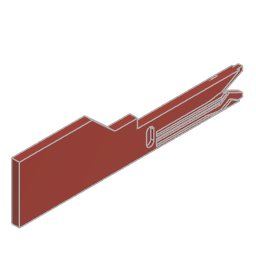
3ks+ finished (Autodesk Fusion 360 design; units mm, degrees)
Autodesk Fusion 360 part; units mm, degrees
note: some values were not read from the file. Set by a fixed rule: which face or edge a step refers to.
sketch "blade" plane through (0, 0, 0) normal (1, 0, 0) x (0, 1, 0)
  line L0 (0, 0) -> (0, 0.75) construction
  line L1 (0, 0.75) -> (25.25, 0.75)
  line L2 (25.25, 0.75) -> (25.25, 8.75)
  line L3 (25.25, 8.75) -> (0, 8.75)
  line L4 (0, 8.75) -> (0, 0.75)
  dimension "d14" = 0.75
  dimension "d15" = 25.25
  dimension "d16" = 8
  constraint coincident L0.start origin
  constraint vertical L0
  constraint horizontal L1
  constraint vertical L2
  constraint horizontal L3
  constraint vertical L4
  measures "d14" distance of L0.start L0.end
  measures "d15" distance of L0.end L1.end
  measures "d16" distance of L0.end L3.end
extrude "Extrude1" add sketch "blade" along normal blind 1.1 makes body 1
sketch "single track" plane through (1.1, 0, 0) normal (1, 0, 0) x (0, 1, 0)
  line L0 (0, 8.75) -> (0, 0.75)
  line L1 (0, 0.75) -> (25.25, 0.75)
  line L2 (25.25, 0.75) -> (25.25, 8.75)
  line L3 (25.25, 8.75) -> (0, 8.75)
  line L4 (0, 0.75) -> (0.9, 0.75) construction
  line L5 (0.9, 0.75) -> (4.4, 0.75) construction
  line L6 (4.4, 0.75) -> (7.9, 0.75) construction
  line L7 (7.9, 0.75) -> (11.4, 0.75) construction
  line L8 (11.4, 0.75) -> (14.9, 0.75) construction
  line L9 (14.9, 0.75) -> (18.4, 0.75) construction
  line L10 (18.4, 0.75) -> (21.9, 0.75) construction
  line L11 (21.9, 0.75) -> (21.9, 4.75) construction
  line L12 (21.9, 4.75) -> (25.25, 4.75)
  line L13 (0.9, 0.75) -> (0.9, 2.75) construction
  line L14 (4.4, 0.75) -> (4.4, 2.75) construction
  line L15 (7.9, 0.75) -> (7.9, 2.75) construction
  line L16 (11.4, 0.75) -> (11.4, 2.75) construction
  line L17 (14.9, 0.75) -> (14.9, 2.75) construction
  line L18 (18.4, 0.75) -> (18.4, 2.75) construction
  circle A0 centre (0.9, 2.75) radius 0.6 construction
  circle A1 centre (4.4, 2.75) radius 0.6 construction
  circle A2 centre (7.9, 2.75) radius 0.6 construction
  circle A3 centre (11.4, 2.75) radius 0.6 construction
  circle A4 centre (14.9, 2.75) radius 0.6 construction
  circle A5 centre (18.4, 2.75) radius 0.6 construction
  line L19 (0.9, 2.75) -> (0, 2.75)
  line L20 (0, 0.75) -> (0, 2.75) construction
  line L21 (0.9, 2.75) -> (1.2, 2.75)
  line L22 (4.4, 2.75) -> (4.1, 2.75)
  line L23 (4.4, 2.75) -> (4.7, 2.75)
  line L24 (7.9, 2.75) -> (7.6, 2.75)
  line L25 (7.9, 2.75) -> (8.2, 2.75)
  line L26 (11.4, 2.75) -> (11.1, 2.75)
  line L27 (11.4, 2.75) -> (11.7, 2.75)
  line L28 (14.9, 2.75) -> (14.6, 2.75)
  line L29 (14.9, 2.75) -> (15.2, 2.75)
  line L30 (18.4, 2.75) -> (18.1, 2.75)
  line L31 (18.4, 2.75) -> (18.7, 2.75)
  line L32 (21.9, 4.75) -> (21.6, 4.75)
  line L33 (1.2, 2.75) -> (4.1, 2.75)
  line L34 (4.7, 2.75) -> (7.6, 2.75)
  line L35 (8.2, 2.75) -> (11.1, 2.75)
  line L36 (11.7, 2.75) -> (14.6, 2.75)
  line L37 (15.2, 2.75) -> (18.1, 2.75)
  line L38 (18.7, 2.75) -> (21.6, 4.75)
  dimension "d19" = 0.9
  dimension "d20" = 3.5
  dimension "d21" = 3.5
  dimension "d22" = 3.5
  dimension "d23" = 3.5
  dimension "d24" = 3.5
  dimension "d25" = 3.5
  dimension "d26" = 2
  dimension "d27" = 2
  dimension "d28" = 2
  dimension "d29" = 2
  dimension "d30" = 2
  dimension "d31" = 2
  dimension "d32" = 1.2
  dimension "d33" = 1.2
  dimension "d34" = 1.2
  dimension "d35" = 1.2
  dimension "d36" = 1.2
  dimension "d37" = 1.2
  dimension "d38" = 0.3
  dimension "d39" = 0.3
  dimension "d40" = 0.3
  dimension "d41" = 0.3
  dimension "d42" = 0.3
  dimension "d43" = 0.3
  dimension "d44" = 0.3
  dimension "d45" = 0.3
  dimension "d46" = 0.3
  dimension "d47" = 0.3
  dimension "d48" = 0.3
  dimension "d49" = 0.3
  constraint coincident L0.end L1.start
  constraint perpendicular L0 L4
  constraint parallel L1 L5
  constraint parallel L1 L6
  constraint parallel L1 L7
  constraint parallel L1 L8
  constraint parallel L1 L9
  constraint parallel L1 L10
  constraint perpendicular L10 L11
  constraint midpoint L2 L12.end
  constraint perpendicular L2 L12
  constraint perpendicular L5 L13
  constraint perpendicular L6 L14
  constraint perpendicular L6 L15
  constraint perpendicular L8 L16
  constraint perpendicular L9 L17
  constraint perpendicular L9 L18
  constraint coincident L13.end A0.centre
  constraint coincident L14.end A1.centre
  constraint coincident L15.end A2.centre
  constraint coincident L16.end A3.centre
  constraint coincident L17.end A4.centre
  constraint coincident L18.end A5.centre
  constraint coincident L0 L19.end
  constraint perpendicular L0 L19
  constraint perpendicular L13 L21
  constraint perpendicular L14 L22
  constraint perpendicular L14 L23
  constraint perpendicular L15 L24
  constraint perpendicular L15 L25
  constraint perpendicular L16 L26
  constraint perpendicular L16 L27
  constraint perpendicular L17 L28
  constraint perpendicular L17 L29
  constraint perpendicular L18 L30
  constraint perpendicular L18 L31
  constraint perpendicular L11 L32
  measures "d19" distance of L0.end L4.end
  measures "d20" distance of L4.end L5.end
  measures "d21" distance of L5.end L6.end
  measures "d22" distance of L6.end L7.end
  measures "d23" distance of L7.end L8.end
  measures "d24" distance of L8.end L9.end
  measures "d25" distance of L9.end L10.end
  measures "d26" distance of L4.end L13.end
  measures "d27" distance of L5.end L14.end
  measures "d28" distance of L6.end L15.end
  measures "d29" distance of L7.end L16.end
  measures "d30" distance of L8.end L17.end
  measures "d31" distance of L9.end L18.end
  measures "d32" diameter of A0
  measures "d33" diameter of A1
  measures "d34" diameter of A2
  measures "d35" diameter of A3
  measures "d36" diameter of A4
  measures "d37" diameter of A5
  measures "d38" distance of L13.end L21.end
  measures "d39" distance of L14.end L22.end
  measures "d40" distance of L14.end L23.end
  measures "d41" distance of L15.end L24.end
  measures "d42" distance of L15.end L25.end
  measures "d43" distance of L16.end L26.end
  measures "d44" distance of L16.end L27.end
  measures "d45" distance of L17.end L28.end
  measures "d46" distance of L17.end L29.end
  measures "d47" distance of L18.end L30.end
  measures "d48" distance of L18.end L31.end
  measures "d49" distance of L11.end L32.end
sketch "single track cutter" plane through (0, 0, 0) normal (0, -1, 0) x (1, 0, 0)
  line L0 (0, 8.75) -> (0, 0.75)
  line L1 (0, 0.75) -> (1.1, 0.75)
  line L2 (1.1, 0.75) -> (1.1, 8.75)
  line L3 (1.1, 8.75) -> (0, 8.75)
  line L4 (1.1, 2.75) -> (1.1, 2.15)
  line L5 (1.1, 2.75) -> (1.1, 3.35)
  line L6 (1.1, 3.35) -> (0.1, 3.35)
  line L7 (0.1, 3.35) -> (0.1, 2.15)
  line L8 (0.1, 2.15) -> (1.1, 2.15)
  point P0 (1.1, 2.75)
  dimension "d50" = 0.6
  dimension "d51" = 0.6
  dimension "d52" = 1
  constraint vertical L4
  constraint coincident P0 L4.start
  constraint parallel L2 L5
  constraint perpendicular L5 L6
  constraint perpendicular L6 L7
  constraint perpendicular L4 L8
  measures "d50" distance of P0 L4.end
  measures "d51" distance of P0 L5.end
  measures "d52" distance of L5.end L6.end
sketch "double track" plane through (1.1, 0, 0) normal (1, 0, 0) x (0, 1, 0)
  line L0 (0, 8.75) -> (0, 0.75)
  line L1 (0, 0.75) -> (25.25, 0.75)
  line L2 (25.25, 0.75) -> (25.25, 8.75)
  line L3 (25.25, 8.75) -> (0, 8.75)
  line L4 (0, 0.75) -> (0.9, 0.75) construction
  line L5 (0.9, 0.75) -> (4.4, 0.75) construction
  line L6 (4.4, 0.75) -> (7.9, 0.75) construction
  line L7 (7.9, 0.75) -> (11.4, 0.75) construction
  line L8 (11.4, 0.75) -> (14.9, 0.75) construction
  line L9 (14.9, 0.75) -> (18.4, 0.75) construction
  line L10 (18.4, 0.75) -> (21.9, 0.75) construction
  line L11 (21.9, 0.75) -> (21.9, 4.75) construction
  line L12 (21.9, 4.75) -> (25.25, 4.75) construction
  line L13 (0.9, 0.75) -> (0.9, 3.25) construction
  line L14 (4.4, 0.75) -> (4.4, 3.25) construction
  line L15 (7.9, 0.75) -> (7.9, 3.25) construction
  line L16 (11.4, 0.75) -> (11.4, 3.25) construction
  line L17 (14.9, 0.75) -> (14.9, 3.25) construction
  line L18 (18.4, 0.75) -> (18.4, 3.25) construction
  line L19 (0.9, 3.25) -> (0.9, 2) construction
  line L20 (0.9, 3.25) -> (0.9, 4.5) construction
  line L21 (4.4, 3.25) -> (4.4, 2) construction
  line L22 (4.4, 3.25) -> (4.4, 4.5) construction
  line L23 (7.9, 3.25) -> (7.9, 2) construction
  line L24 (7.9, 3.25) -> (7.9, 4.5) construction
  line L25 (11.4, 3.25) -> (11.4, 2) construction
  line L26 (11.4, 3.25) -> (11.4, 4.5) construction
  line L27 (14.9, 3.25) -> (14.9, 2) construction
  line L28 (14.9, 3.25) -> (14.9, 4.5) construction
  line L29 (18.4, 3.25) -> (18.4, 1.75) construction
  line L30 (18.4, 3.25) -> (18.4, 4.75) construction
  circle A0 centre (0.9, 2) radius 0.6 construction
  circle A1 centre (0.9, 4.5) radius 0.6 construction
  circle A2 centre (4.4, 2) radius 0.6 construction
  circle A3 centre (4.4, 4.5) radius 0.6 construction
  circle A4 centre (7.9, 2) radius 0.6 construction
  circle A5 centre (7.9, 4.5) radius 0.6 construction
  circle A6 centre (11.4, 2) radius 0.6 construction
  circle A7 centre (11.4, 4.5) radius 0.6 construction
  circle A8 centre (14.9, 2) radius 0.6 construction
  circle A9 centre (14.9, 4.5) radius 0.6 construction
  circle A10 centre (18.4, 1.75) radius 0.85 construction
  circle A11 centre (18.4, 4.75) radius 0.85 construction
  line L31 (0.9, 2) -> (0, 2)
  line L32 (0.9, 4.5) -> (0, 4.5)
  line L33 (0, 0.75) -> (0, 2) construction
  line L34 (0, 0.75) -> (0, 4.5) construction
  line L35 (0.9, 2) -> (1.2, 2)
  line L36 (4.4, 2) -> (4.1, 2)
  line L37 (4.4, 2) -> (4.7, 2)
  line L38 (7.9, 2) -> (7.6, 2)
  line L39 (7.9, 2) -> (8.2, 2)
  line L40 (11.4, 2) -> (11.1, 2)
  line L41 (11.4, 2) -> (11.7, 2)
  line L42 (14.9, 2) -> (14.6, 2)
  line L43 (14.9, 2) -> (15.2, 2)
  line L44 (18.4, 1.75) -> (18.1, 1.75)
  line L45 (18.4, 1.75) -> (18.7, 1.75)
  line L46 (21.9, 4.75) -> (21.9, 3.25) construction
  line L47 (21.9, 4.75) -> (21.9, 6.25) construction
  line L48 (21.9, 3.25) -> (21.6, 3.25) construction
  line L49 (0.9, 4.5) -> (1.2, 4.5)
  line L50 (4.4, 4.5) -> (4.1, 4.5)
  line L51 (4.4, 4.5) -> (4.7, 4.5)
  line L52 (7.9, 4.5) -> (7.6, 4.5)
  line L53 (7.9, 4.5) -> (8.2, 4.5)
  line L54 (11.4, 4.5) -> (11.1, 4.5)
  line L55 (11.4, 4.5) -> (11.7, 4.5)
  line L56 (14.9, 4.5) -> (14.6, 4.5)
  line L57 (14.9, 4.5) -> (15.2, 4.5)
  line L58 (18.4, 4.75) -> (18.1, 4.75)
  line L59 (18.4, 4.75) -> (18.7, 4.75)
  line L60 (21.9, 6.25) -> (21.6, 6.25) construction
  line L61 (1.2, 2) -> (4.1, 2)
  line L62 (4.7, 2) -> (7.6, 2)
  line L63 (8.2, 2) -> (11.1, 2)
  line L64 (11.7, 2) -> (14.6, 2)
  line L65 (15.2, 2) -> (18.1, 1.75)
  line L66 (18.7, 1.75) -> (21.6, 3.25)
  line L67 (21.6, 3.25) -> (25.25, 1.0914)
  line L68 (21.6, 3.25) -> (25.25, 3.25) construction
  line L69 (25.25, 1.0914) -> (26.3259, 0.4551)
  line L70 (1.2, 4.5) -> (4.1, 4.5)
  line L71 (4.7, 4.5) -> (7.6, 4.5)
  line L72 (8.2, 4.5) -> (11.1, 4.5)
  line L73 (11.7, 4.5) -> (14.6, 4.5)
  line L74 (15.2, 4.5) -> (18.1, 4.75)
  line L75 (18.7, 4.75) -> (21.6, 6.25)
  line L76 (21.6, 6.25) -> (25.25, 8.4086)
  line L77 (21.6, 6.25) -> (25.25, 6.25) construction
  line L78 (25.25, 8.4086) -> (26.3259, 9.0449)
  dimension "d53" = 0.9
  dimension "d54" = 3.5
  dimension "d55" = 3.5
  dimension "d56" = 3.5
  dimension "d57" = 3.5
  dimension "d58" = 3.5
  dimension "d59" = 3.5
  dimension "d60" = 2.5
  dimension "d61" = 2.5
  dimension "d62" = 2.5
  dimension "d63" = 2.5
  dimension "d64" = 2.5
  dimension "d65" = 2.5
  dimension "d66" = 1.25
  dimension "d67" = 1.25
  dimension "d68" = 1.25
  dimension "d69" = 1.25
  dimension "d70" = 1.25
  dimension "d71" = 1.25
  dimension "d72" = 1.25
  dimension "d73" = 1.25
  dimension "d74" = 1.25
  dimension "d75" = 1.25
  dimension "d77" = 1.5
  dimension "d78" = 1.5
  dimension "d79" = 1.2
  dimension "d80" = 1.2
  dimension "d81" = 1.2
  dimension "d82" = 1.2
  dimension "d83" = 1.2
  dimension "d84" = 1.2
  dimension "d85" = 1.2
  dimension "d86" = 1.2
  dimension "d87" = 1.2
  dimension "d88" = 1.2
  dimension "d89" = 1.7
  dimension "d90" = 1.7
  dimension "d91" = 0.3
  dimension "d92" = 0.3
  dimension "d93" = 0.3
  dimension "d94" = 0.3
  dimension "d95" = 0.3
  dimension "d96" = 0.3
  dimension "d97" = 0.3
  dimension "d98" = 0.3
  dimension "d99" = 0.3
  dimension "d100" = 0.3
  dimension "d101" = 0.3
  dimension "d102" = 1.5
  dimension "d103" = 1.5
  dimension "d104" = 0.3
  dimension "d105" = 0.3
  dimension "d106" = 0.3
  dimension "d107" = 0.3
  dimension "d108" = 0.3
  dimension "d109" = 0.3
  dimension "d110" = 0.3
  dimension "d111" = 0.3
  dimension "d112" = 0.3
  dimension "d113" = 0.3
  dimension "d114" = 0.3
  dimension "d115" = 0.3
  dimension "d116" = 0.3
  dimension "d117" = 149.4
  dimension "d118" = 1.25
  dimension "d119" = 149.4
  dimension "d120" = 1.25
  constraint coincident L0.end L1.start
  constraint perpendicular L0 L4
  constraint parallel L1 L5
  constraint parallel L1 L6
  constraint parallel L1 L7
  constraint parallel L1 L8
  constraint parallel L1 L9
  constraint parallel L1 L10
  constraint perpendicular L10 L11
  constraint midpoint L2 L12.end
  constraint perpendicular L2 L12
  constraint perpendicular L4 L13
  constraint perpendicular L6 L14
  constraint perpendicular L7 L15
  constraint perpendicular L7 L16
  constraint perpendicular L8 L17
  constraint perpendicular L9 L18
  constraint parallel L13 L19
  constraint parallel L19 L20
  constraint parallel L14 L21
  constraint parallel L14 L22
  constraint parallel L15 L23
  constraint parallel L15 L24
  constraint parallel L16 L25
  constraint parallel L25 L26
  constraint parallel L17 L27
  constraint parallel L27 L28
  constraint parallel L18 L29
  constraint parallel L29 L30
  constraint coincident L19.end A0.centre
  constraint coincident L20.end A1.centre
  constraint coincident L21.end A2.centre
  constraint coincident L22.end A3.centre
  constraint coincident L23.end A4.centre
  constraint coincident L24.end A5.centre
  constraint coincident L25.end A6.centre
  constraint coincident L26.end A7.centre
  constraint coincident L27.end A8.centre
  constraint coincident L28.end A9.centre
  constraint coincident L29.end A10.centre
  constraint coincident L30.end A11.centre
  constraint coincident L0 L31.end
  constraint perpendicular L0 L31
  constraint coincident L0 L32.end
  constraint perpendicular L0 L32
  constraint perpendicular L19 L35
  constraint perpendicular L14 L36
  constraint perpendicular L21 L37
  constraint perpendicular L15 L38
  constraint perpendicular L15 L39
  constraint perpendicular L16 L40
  constraint perpendicular L25 L41
  constraint perpendicular L27 L42
  constraint perpendicular L17 L43
  constraint perpendicular L18 L44
  constraint perpendicular L29 L45
  constraint perpendicular L12 L46
  constraint perpendicular L12 L47
  constraint perpendicular L46 L48
  constraint perpendicular L20 L49
  constraint perpendicular L22 L50
  constraint perpendicular L22 L51
  constraint perpendicular L24 L52
  constraint perpendicular L24 L53
  constraint perpendicular L26 L54
  constraint perpendicular L26 L55
  constraint perpendicular L28 L56
  constraint perpendicular L28 L57
  constraint perpendicular L30 L58
  constraint perpendicular L30 L59
  constraint perpendicular L47 L60
  constraint horizontal L68
  constraint coincident L2 L67.end
  constraint coincident L2 L68.end
  constraint parallel L67 L69
  constraint horizontal L77
  constraint coincident L2 L76.end
  constraint coincident L2 L77.end
  constraint parallel L76 L78
  measures "d53" distance of L0.end L4.end
  measures "d54" distance of L4.end L5.end
  measures "d55" distance of L5.end L6.end
  measures "d56" distance of L6.end L7.end
  measures "d57" distance of L7.end L8.end
  measures "d58" distance of L8.end L9.end
  measures "d59" distance of L9.end L10.end
  measures "d60" distance of L4.end L13.end
  measures "d61" distance of L5.end L14.end
  measures "d62" distance of L6.end L15.end
  measures "d63" distance of L7.end L16.end
  measures "d64" distance of L8.end L17.end
  measures "d65" distance of L9.end L18.end
  measures "d66" distance of L13.end L19.end
  measures "d67" distance of L13.end L20.end
  measures "d68" distance of L14.end L21.end
  measures "d69" distance of L14.end L22.end
  measures "d70" distance of L15.end L23.end
  measures "d71" distance of L15.end L24.end
  measures "d72" distance of L16.end L25.end
  measures "d73" distance of L16.end L26.end
  measures "d74" distance of L17.end L27.end
  measures "d75" distance of L17.end L28.end
  measures "d77" distance of L18.end L29.end
  measures "d78" distance of L18.end L30.end
  measures "d79" diameter of A0
  measures "d80" diameter of A1
  measures "d81" diameter of A2
  measures "d82" diameter of A3
  measures "d83" diameter of A4
  measures "d84" diameter of A5
  measures "d85" diameter of A6
  measures "d86" diameter of A7
  measures "d87" diameter of A8
  measures "d88" diameter of A9
  measures "d89" diameter of A10
  measures "d90" diameter of A11
  measures "d91" distance of L19.end L35.end
  measures "d92" distance of L21.end L36.end
  measures "d93" distance of L21.end L37.end
  measures "d94" distance of L23.end L38.end
  measures "d95" distance of L23.end L39.end
  measures "d96" distance of L25.end L40.end
  measures "d97" distance of L25.end L41.end
  measures "d98" distance of L27.end L42.end
  measures "d99" distance of L27.end L43.end
  measures "d100" distance of L29.end L44.end
  measures "d101" distance of L29.end L45.end
  measures "d102" distance of L11.end L46.end
  measures "d103" distance of L11.end L47.end
  measures "d104" distance of L46.end L48.end
  measures "d105" distance of L20.end L49.end
  measures "d106" distance of L22.end L50.end
  measures "d107" distance of L22.end L51.end
  measures "d108" distance of L24.end L52.end
  measures "d109" distance of L24.end L53.end
  measures "d110" distance of L26.end L54.end
  measures "d111" distance of L26.end L55.end
  measures "d112" distance of L28.end L56.end
  measures "d113" distance of L28.end L57.end
  measures "d114" distance of L30.end L58.end
  measures "d115" distance of L30.end L59.end
  measures "d116" distance of L47.end L60.end
  measures "d117" angle of L67 L68
  measures "d118" distance of L67.end L69.end
  measures "d119" angle of L76 L77
  measures "d120" distance of L76.end L78.end
sketch "double track cutter" plane through (0, 0, 0) normal (0, -1, 0) x (1, 0, 0)
  line L0 (0, 8.75) -> (0, 0.75)
  line L1 (0, 0.75) -> (1.1, 0.75)
  line L2 (1.1, 0.75) -> (1.1, 8.75)
  line L3 (1.1, 8.75) -> (0, 8.75)
  line L4 (1.1, 2) -> (1.1, 1.4)
  line L5 (1.1, 4.5) -> (1.1, 3.9)
  line L6 (1.1, 2) -> (1.1, 2.6)
  line L7 (1.1, 4.5) -> (1.1, 5.1)
  line L8 (1.1, 1.4) -> (0.6, 1.4)
  line L9 (1.1, 5.1) -> (0.6, 5.1)
  line L10 (0.6, 1.4) -> (0.6, 2.6)
  line L11 (0.6, 2.6) -> (1.1, 2.6)
  line L12 (0.6, 5.1) -> (0.6, 3.9)
  line L13 (0.6, 3.9) -> (1.1, 3.9)
  point P0 (1.1, 2)
  point P1 (1.1, 4.5)
  dimension "d121" = 0.6
  dimension "d122" = 0.6
  dimension "d123" = 0.6
  dimension "d124" = 0.6
  dimension "d125" = 0.5
  dimension "d126" = 0.5
  constraint vertical L4
  constraint coincident P0 L4.start
  constraint vertical L5
  constraint coincident P1 L5.start
  constraint parallel L2 L6
  constraint parallel L2 L7
  constraint perpendicular L4 L8
  constraint perpendicular L7 L9
  constraint perpendicular L8 L10
  constraint perpendicular L6 L11
  constraint perpendicular L9 L12
  constraint perpendicular L5 L13
  measures "d121" distance of P0 L4.end
  measures "d122" distance of P1 L5.end
  measures "d123" distance of P0 L6.end
  measures "d124" distance of P1 L7.end
  measures "d125" distance of L4.end L8.end
  measures "d126" distance of L7.end L9.end
sketch "wider double track" plane through (1.1, 0, 0) normal (1, 0, 0) x (0, 1, 0)
  line L0 (0, 8.75) -> (0, 0.75)
  line L1 (0, 0.75) -> (25.25, 0.75)
  line L2 (25.25, 0.75) -> (25.25, 8.75)
  line L3 (25.25, 8.75) -> (0, 8.75)
  line L4 (0, 0.75) -> (14.9, 0.75) construction
  line L5 (14.9, 0.75) -> (18.4, 0.75) construction
  line L6 (18.4, 0.75) -> (21.9, 0.75) construction
  line L7 (14.9, 0.75) -> (14.9, 3.25) construction
  line L8 (18.4, 0.75) -> (18.4, 3.25) construction
  line L9 (21.9, 0.75) -> (21.9, 4.75) construction
  line L10 (21.9, 4.75) -> (25.25, 4.75) construction
  line L11 (14.9, 3.25) -> (14.9, 2) construction
  line L12 (14.9, 3.25) -> (14.9, 4.5) construction
  line L13 (14.9, 2) -> (14.9, 1.4) construction
  line L14 (14.9, 2) -> (14.9, 2.6) construction
  line L15 (14.9, 2) -> (14.3, 2) construction
  line L16 (14.9, 4.5) -> (14.9, 3.9) construction
  line L17 (14.9, 4.5) -> (14.3, 4.5) construction
  line L18 (14.9, 4.5) -> (14.9, 5.1) construction
  arc A0 (14.9, 2.6) -> (14.9, 1.4) centre (14.9, 2) ccw
  arc A1 (14.9, 5.1) -> (14.9, 3.9) centre (14.9, 4.5) ccw
  line L19 (14.9, 5.1) -> (15.2, 5.1)
  line L20 (14.9, 3.9) -> (15.2, 3.9)
  line L21 (14.9, 1.4) -> (15.2, 1.4)
  line L22 (14.9, 2.6) -> (15.2, 2.6)
  line L23 (18.4, 3.25) -> (18.4, 1.75) construction
  line L24 (18.4, 3.25) -> (18.4, 4.75) construction
  line L25 (18.4, 1.75) -> (18.15, 1.5) construction
  line L26 (18.4, 1.75) -> (18.175, 1.75) construction
  line L27 (18.4, 1.75) -> (18.15, 2) construction
  line L28 (18.4, 1.75) -> (18.175, 1.75) construction
  line L29 (18.4, 1.75) -> (18.175, 1.75) construction
  line L30 (18.4, 4.75) -> (18.15, 4.5) construction
  line L31 (18.4, 4.75) -> (18.175, 4.75) construction
  line L32 (18.4, 4.75) -> (18.15, 5) construction
  line L33 (18.4, 4.75) -> (18.175, 4.75) construction
  line L34 (18.4, 4.75) -> (18.175, 4.75) construction
  line L35 (18.15, 1.5) -> (18.15, 0.9) construction
  line L36 (18.15, 0.9) -> (17.85, 0.9)
  line L37 (17.85, 0.9) -> (15.2, 1.4)
  line L38 (21.9, 4.75) -> (21.9, 3.25) construction
  line L39 (21.9, 4.75) -> (21.9, 6.25) construction
  line L40 (21.9, 3.25) -> (21.6, 3.25) construction
  line L41 (21.9, 6.25) -> (21.6, 6.25) construction
  line L42 (21.6, 3.25) -> (25.25, 1.0914)
  line L43 (21.6, 3.25) -> (25.25, 3.25) construction
  line L44 (25.25, 1.0914) -> (26.5411, 0.3278)
  line L45 (26.5411, 0.3278) -> (28.0411, 0.3278)
  line L46 (18.15, 2) -> (18.15, 2.6) construction
  line L47 (18.15, 2) -> (18.75, 2) construction
  line L48 (18.15, 1.5) -> (18.75, 1.5) construction
  line L49 (18.4, 1.75) -> (18.6954, 1.75) construction
  arc A2 (18.6954, 1.75) -> (18.15, 2.6) centre (18.15, 2) ccw
  arc A3 (18.15, 0.9) -> (18.6954, 1.75) centre (18.15, 1.5) ccw
  line L50 (18.15, 2.6) -> (17.85, 2.6)
  line L51 (17.85, 2.6) -> (15.2, 2.6)
  line L52 (18.4, 1.75) -> (18.825, 1.75)
  line L53 (18.825, 1.75) -> (21.6, 3.25)
  line L54 (18.4, 1.75) -> (18.15, 1.75)
  line L55 (18.15, 4.5) -> (18.15, 3.9) construction
  line L56 (18.15, 4.5) -> (18.75, 4.5) construction
  line L57 (18.15, 5) -> (18.15, 5.6) construction
  line L58 (18.15, 5) -> (18.75, 5) construction
  line L59 (18.4, 4.75) -> (18.6954, 4.75) construction
  arc A4 (18.6954, 4.75) -> (18.15, 5.6) centre (18.15, 5) ccw
  arc A5 (18.15, 3.9) -> (18.6954, 4.75) centre (18.15, 4.5) ccw
  line L60 (18.15, 3.9) -> (17.85, 3.9)
  line L61 (18.15, 5.6) -> (17.85, 5.6)
  line L62 (17.85, 5.6) -> (15.2, 5.1)
  line L63 (15.2, 3.9) -> (17.85, 3.9)
  line L64 (18.4, 4.75) -> (18.825, 4.75)
  line L65 (18.4, 4.75) -> (18.15, 4.75)
  line L66 (21.6, 6.25) -> (25.25, 8.4086)
  line L67 (21.6, 6.25) -> (25.25, 6.25) construction
  line L68 (25.25, 8.4086) -> (26.5411, 9.1722)
  line L69 (26.5411, 9.1722) -> (28.0411, 9.1722)
  line L70 (21.6, 6.25) -> (18.825, 4.75)
  dimension "d127" = 14.9
  dimension "d128" = 3.5
  dimension "d129" = 3.5
  dimension "d130" = 2.5
  dimension "d131" = 2.5
  dimension "d132" = 1.25
  dimension "d133" = 1.25
  dimension "d134" = 0.6
  dimension "d135" = 0.6
  dimension "d136" = 0.6
  dimension "d137" = 0.6
  dimension "d138" = 0.6
  dimension "d139" = 0.6
  dimension "d140" = 0.3
  dimension "d141" = 0.3
  dimension "d142" = 0.3
  dimension "d143" = 0.3
  dimension "d144" = 1.5
  dimension "d145" = 1.5
  dimension "d146" = 45
  dimension "d147" = 0.3536
  dimension "d148" = 45
  dimension "d149" = 0.3536
  dimension "d150" = 0.225
  dimension "d151" = 45
  dimension "d152" = 0.3536
  dimension "d153" = 45
  dimension "d154" = 0.3536
  dimension "d155" = 0.225
  dimension "d156" = 0.6
  dimension "d162" = 0.3
  dimension "d165" = 1.5
  dimension "d166" = 1.5
  dimension "d167" = 0.3
  dimension "d168" = 0.3
  dimension "d169" = 149.4
  dimension "d170" = 1.5
  dimension "d171" = 1.5
  dimension "d172" = 0.6
  dimension "d173" = 0.6
  dimension "d174" = 0.6
  dimension "d175" = 0.3
  dimension "d176" = 0.425
  dimension "d177" = 0.25
  dimension "d178" = 0.6
  dimension "d179" = 0.6
  dimension "d180" = 0.6
  dimension "d181" = 0.6
  dimension "d182" = 0.3
  dimension "d183" = 0.3
  dimension "d184" = 0.425
  dimension "d185" = 0.25
  dimension "d186" = 149.4
  dimension "d187" = 1.5
  dimension "d188" = 1.5
  constraint coincident L0.end L1.start
  constraint perpendicular L0 L4
  constraint parallel L1 L5
  constraint parallel L1 L6
  constraint perpendicular L4 L7
  constraint perpendicular L1 L8
  constraint perpendicular L6 L9
  constraint midpoint L2 L10.end
  constraint perpendicular L2 L10
  constraint parallel L7 L11
  constraint parallel L11 L12
  constraint perpendicular L5 L13
  constraint parallel L7 L14
  constraint perpendicular L13 L15
  constraint parallel L12 L16
  constraint perpendicular L16 L17
  constraint perpendicular L17 L18
  constraint coincident L15.end A0
  constraint coincident L17.end A1
  constraint perpendicular L18 L19
  constraint perpendicular L12 L20
  constraint perpendicular L7 L21
  constraint perpendicular L11 L22
  constraint parallel L8 L23
  constraint parallel L23 L24
  constraint horizontal L26
  constraint horizontal L28
  constraint perpendicular L23 L29
  constraint horizontal L31
  constraint horizontal L33
  constraint perpendicular L24 L34
  constraint parallel L8 L35
  constraint perpendicular L35 L36
  constraint perpendicular L10 L38
  constraint perpendicular L10 L39
  constraint perpendicular L9 L40
  constraint perpendicular L39 L41
  constraint horizontal L43
  constraint coincident L2 L42.end
  constraint coincident L2 L43.end
  constraint parallel L42 L44
  constraint horizontal L45
  constraint parallel L8 L46
  constraint perpendicular L46 L47
  constraint perpendicular L35 L48
  constraint perpendicular L23 L49
  constraint coincident L49 A2.start
  constraint coincident L27.end L46.start
  constraint coincident L49.end A2.start
  constraint coincident L25 L35.start
  constraint perpendicular L46 L50
  constraint perpendicular L8 L52
  constraint perpendicular L23 L54
  constraint parallel L24 L55
  constraint perpendicular L55 L56
  constraint perpendicular L56 L57
  constraint perpendicular L57 L58
  constraint perpendicular L24 L59
  constraint coincident L59 A4.start
  constraint coincident L32.end L57.start
  constraint coincident L59.end A4.start
  constraint coincident L30 L55.start
  constraint perpendicular L55 L60
  constraint perpendicular L57 L61
  constraint perpendicular L24 L64
  constraint perpendicular L24 L65
  constraint horizontal L67
  constraint coincident L2 L66.end
  constraint coincident L2 L67.end
  constraint parallel L66 L68
  constraint horizontal L69
  measures "d127" distance of L0.end L4.end
  measures "d128" distance of L4.end L5.end
  measures "d129" distance of L5.end L6.end
  measures "d130" distance of L4.end L7.end
  measures "d131" distance of L5.end L8.end
  measures "d132" distance of L7.end L11.end
  measures "d133" distance of L7.end L12.end
  measures "d134" distance of L11.end L13.end
  measures "d135" distance of L11.end L14.end
  measures "d136" distance of L11.end L15.end
  measures "d137" distance of L12.end L16.end
  measures "d138" distance of L12.end L17.end
  measures "d139" distance of L12.end L18.end
  measures "d140" distance of L18.end L19.end
  measures "d141" distance of L16.end L20.end
  measures "d142" distance of L13.end L21.end
  measures "d143" distance of L14.end L22.end
  measures "d144" distance of L8.end L23.end
  measures "d145" distance of L8.end L24.end
  measures "d146" angle of L25 L26
  measures "d147" distance of L23.end L25.end
  measures "d148" angle of L27 L28
  measures "d149" distance of L23.end L27.end
  measures "d150" distance of L23.end L26.end
  measures "d151" angle of L30 L31
  measures "d152" distance of L24.end L30.end
  measures "d153" angle of L32 L33
  measures "d154" distance of L24.end L32.end
  measures "d155" distance of L24.end L31.end
  measures "d156" distance of L25.end L35.end
  measures "d162" distance of L35.end L36.end
  measures "d165" distance of L9.end L38.end
  measures "d166" distance of L9.end L39.end
  measures "d167" distance of L38.end L40.end
  measures "d168" distance of L39.end L41.end
  measures "d169" angle of L42 L43
  measures "d170" distance of L42.end L44.end
  measures "d171" distance of L44.end L45.end
  measures "d172" distance of L27.end L46.end
  measures "d173" distance of L27.end L47.end
  measures "d174" distance of L25.end L48.end
  measures "d175" distance of L46.end L50.end
  measures "d176" distance of L23.end L52.end
  measures "d177" distance of L23.end L54.end
  measures "d178" distance of L30.end L55.end
  measures "d179" distance of L30.end L56.end
  measures "d180" distance of L32.end L57.end
  measures "d181" distance of L32.end L58.end
  measures "d182" distance of L55.end L60.end
  measures "d183" distance of L57.end L61.end
  measures "d184" distance of L24.end L64.end
  measures "d185" distance of L24.end L65.end
  measures "d186" angle of L66 L67
  measures "d187" distance of L66.end L68.end
  measures "d188" distance of L68.end L69.end
ref_plane "WorkPlane1" through (0.55, 28.0411, 4.75) normal (0, 1, 0) x (0, 0, 1)
sketch "wider double track cutter" plane through (0, 28.0411, 0) normal (0, 1, 0) x (1, 0, 0)
  line L0 (1.1, -9.1722) -> (1.1, -10.0222)
  line L1 (1.1, -0.3278) -> (1.1, 0.5222)
  line L2 (1.1, -0.3278) -> (1.1, -1.1778)
  line L3 (1.1, -9.1722) -> (1.1, -8.3222)
  line L4 (1.1, -10.0222) -> (0.6, -10.0222)
  line L5 (1.1, 0.5222) -> (0.6, 0.5222)
  line L6 (0.6, 0.5222) -> (0.6, -1.1778)
  line L7 (0.6, -1.1778) -> (1.1, -1.1778)
  line L8 (0.6, -10.0222) -> (0.6, -8.3222)
  line L9 (0.6, -8.3222) -> (1.1, -8.3222)
  point P0 (1.1, -9.1722)
  point P1 (1.1, -0.3278)
  dimension "d190" = 0.85
  dimension "d191" = 0.85
  dimension "d192" = 0.85
  dimension "d193" = 0.85
  dimension "d194" = 0.5
  dimension "d195" = 0.5
  constraint vertical L0
  constraint coincident P0 L0.start
  constraint vertical L1
  constraint coincident P1 L1.start
  constraint parallel L1 L2
  constraint parallel L0 L3
  constraint perpendicular L0 L4
  constraint perpendicular L1 L5
  constraint perpendicular L5 L6
  constraint perpendicular L2 L7
  constraint perpendicular L4 L8
  constraint perpendicular L3 L9
  measures "d190" distance of P0 L0.end
  measures "d191" distance of P1 L1.end
  measures "d192" distance of P1 L2.end
  measures "d193" distance of P0 L3.end
  measures "d194" distance of L0.end L4.end
  measures "d195" distance of L1.end L5.end
extrude "sidebar hole extension" add 1 faces at (0.3667, 0, 6.0833) along direction (0, -1, 0) blind 5.5 on bodies 1 bodies 1
sketch "sidebar hole" plane through (1.1, 0, 0) normal (1, 0, 0) x (0, 1, 0)
  line L0 (-5.5, 0.75) -> (25.25, 0.75)
  line L1 (25.25, 0.75) -> (25.25, 8.75)
  line L2 (25.25, 8.75) -> (-5.5, 8.75)
  line L3 (-5.5, 8.75) -> (-5.5, 0.75)
  line L4 (-5.5, 0.75) -> (0, 0.75) construction
  line L5 (0, 0.75) -> (0, 4.75) construction
  line L6 (0, 4.75) -> (-2.9, 4.75) construction
  line L7 (-2.9, 4.75) -> (-2.9, 3.3)
  line L8 (-2.9, 3.3) -> (-2.9, 2.25) construction
  line L9 (-2.9, 2.25) -> (-0.8, 2.25) construction
  line L10 (-0.8, 2.25) -> (-0.8, 3.3) construction
  line L11 (-2.9, 4.75) -> (-2.9, 6.2)
  line L12 (-2.9, 6.2) -> (-2.9, 7.25) construction
  line L13 (-2.9, 7.25) -> (-0.8, 7.25) construction
  line L14 (-0.8, 7.25) -> (-0.8, 6.2) construction
  line L15 (-0.8, 6.2) -> (-0.8, 3.3)
  arc A0 (-0.8, 6.2) -> (-2.9, 6.2) centre (-1.85, 6.2) ccw
  arc A1 (-2.9, 3.3) -> (-0.8, 3.3) centre (-1.85, 3.3) ccw
  dimension "d198" = 5.5
  dimension "d199" = 4
  dimension "d200" = 2.9
  dimension "d201" = 1.45
  dimension "d202" = 1.05
  dimension "d203" = 2.1
  dimension "d204" = 1.05
  dimension "d205" = 1.45
  dimension "d206" = 1.05
  dimension "d207" = 2.1
  dimension "d208" = 1.05
  constraint coincident L0.start L3.end
  constraint perpendicular L3 L4
  constraint perpendicular L4 L5
  constraint perpendicular L5 L6
  constraint perpendicular L6 L7
  constraint parallel L7 L8
  constraint perpendicular L8 L9
  constraint perpendicular L9 L10
  constraint perpendicular L6 L11
  constraint perpendicular L6 L12
  constraint perpendicular L12 L13
  constraint perpendicular L13 L14
  constraint tangent L13 A0
  constraint tangent L9 A1
  measures "d198" distance of L0.start L4.end
  measures "d199" distance of L4.end L5.end
  measures "d200" distance of L5.end L6.end
  measures "d201" distance of L6.end L7.end
  measures "d202" distance of L7.end L8.end
  measures "d203" distance of L8.end L9.end
  measures "d204" distance of L9.end L10.end
  measures "d205" distance of L6.end L11.end
  measures "d206" distance of L11.end L12.end
  measures "d207" distance of L12.end L13.end
  measures "d208" distance of L13.end L14.end
sketch "feed ramp" plane through (1.1, 0, 0) normal (1, 0, 0) x (0, 1, 0)
  line L0 (-5.5, 0.75) -> (25.25, 0.75)
  line L1 (25.25, 0.75) -> (25.25, 8.75)
  line L2 (25.25, 8.75) -> (-5.5, 8.75)
  line L3 (-5.5, 8.75) -> (-5.5, 0.75)
  line L4 (25.25, 0.75) -> (25.25, 4.75) construction
  line L5 (25.25, 4.75) -> (21.9, 4.75) construction
  line L6 (21.9, 4.75) -> (21.9, 6) construction
  line L7 (21.9, 4.75) -> (21.9, 3.5) construction
  line L8 (21.9, 6) -> (22.2, 6) construction
  line L9 (21.9, 3.5) -> (22.2, 3.5) construction
  line L10 (22.2, 3.5) -> (25.25, 2.0124)
  line L11 (22.2, 3.5) -> (25.25, 3.5) construction
  line L12 (22.2, 6) -> (25.25, 7.4876)
  line L13 (22.2, 6) -> (25.25, 6) construction
  line L14 (22.2, 6) -> (19.6371, 4.75)
  line L15 (22.2, 3.5) -> (19.6371, 4.75)
  dimension "d209" = 3.35
  dimension "d210" = 1.25
  dimension "d211" = 1.25
  dimension "d212" = 0.3
  dimension "d213" = 0.3
  dimension "d214" = 154
  dimension "d215" = 154
  constraint coincident L0.end L1.start
  constraint midpoint L1 L4.end
  constraint perpendicular L4 L5
  constraint perpendicular L5 L6
  constraint perpendicular L5 L7
  constraint perpendicular L6 L8
  constraint perpendicular L7 L9
  constraint horizontal L11
  constraint coincident L4 L10.end
  constraint coincident L4 L11.end
  constraint horizontal L13
  constraint coincident L1 L12.end
  constraint coincident L1 L13.end
  constraint parallel L12 L14
  constraint coincident L14 L15.end
  constraint parallel L10 L15
  constraint coincident L14.end L15.end
  measures "d209" distance of L4.end L5.end
  measures "d210" distance of L5.end L6.end
  measures "d211" distance of L5.end L7.end
  measures "d212" distance of L6.end L8.end
  measures "d213" distance of L7.end L9.end
  measures "d214" angle of L10 L11
  measures "d215" angle of L12 L13
sketch "bow" plane through (1.1, 0, 0) normal (1, 0, 0) x (0, 1, 0)
  line L0 (-5.5, 0.75) -> (25.25, 0.75)
  line L1 (25.25, 0.75) -> (25.25, 8.75)
  line L2 (25.25, 8.75) -> (-5.5, 8.75)
  line L3 (-5.5, 8.75) -> (-5.5, 0.75)
  line L4 (-5.5, 0.75) -> (-39.5, 0.75)
  line L5 (-39.5, 0.75) -> (-39.5, 17.25)
  line L6 (-39.5, 17.25) -> (-18.5, 17.25)
  line L7 (-5.5, 8.75) -> (-5.5, 11.25)
  line L8 (-5.5, 11.25) -> (-12, 11.25)
  line L9 (-12, 11.25) -> (-18.5, 17.25)
  dimension "d216" = 34
  dimension "d217" = 16.5
  dimension "d218" = 21
  dimension "d219" = 2.5
  dimension "d220" = 6.5
  constraint coincident L0.start L3.end
  constraint perpendicular L3 L4
  constraint perpendicular L4 L5
  constraint perpendicular L5 L6
  constraint coincident L2.end L3.start
  constraint perpendicular L2 L7
  constraint perpendicular L7 L8
  measures "d216" distance of L0.start L4.end
  measures "d217" distance of L4.end L5.end
  measures "d218" distance of L5.end L6.end
  measures "d219" distance of L2.end L7.end
  measures "d220" distance of L7.end L8.end
extrude "Extrude3" cut sketch "sidebar hole" against normal blind 0.85 contours L7 L11 L15 A0 A1 bodies 1
extrude "Extrude4" cut sketch "feed ramp" against normal blind 1.1 contours L1 L10 L12 L14 L15 bodies 1
extrude "Extrude5" cut sketch "wider double track" against normal blind 0.5 contours A0 L21 L22 L36 L37 A2 A3 L50 L51 | A1 L19 L20 A4 A5 L60 L61 L62 L63 bodies 1
sweep "Sweep1" cut profiles "wider double track cutter" path "wider double track" along L54 L52 L53 L42 L44 L45 section 1 contours L1 L2 L5 L6 L7 bodies 1
sweep "Sweep2" cut profiles "wider double track cutter" path "wider double track" along L65 L64 L70 L66 L68 L69 section 1 contours L0 L3 L4 L8 L9 bodies 1
sweep "Sweep3" cut profiles "single track cutter" path "single track" along L12 L32 L38 L31 L30 L37 L29 L28 L36 L27 L26 L35 L25 L24 L34 L23 L22 L33 L21 L19 section 1 contours L2 L4 L5 L6 L7 L8 bodies 1
sweep "Sweep4" cut profiles "double track cutter" path "double track" along L31 L35 L61 L36 L37 L62 L38 L39 L63 L40 L41 L64 L42 L43 L65 L44 L45 L66 L67 L69 section 1 contours L2 L4 L6 L8 L10 L11 bodies 1
sweep "Sweep5" cut profiles "double track cutter" path "double track" along L78 L76 L75 L59 L58 L74 L57 L56 L73 L55 L54 L72 L53 L52 L71 L51 L50 L70 L49 L32 section 1 contours L2 L5 L7 L9 L12 L13 bodies 1
copy_body "CopyPasteBodies1" bodies 1 makes body 2
move_body "Move1" bodies 2 to x (-1, 0, 0) y (0, 1, 0) z (0, 0, -1) at (0, 0, 1.5)
move_body "Move2" bodies 2 to x (1, 0, 0) y (0, 1, 0) z (0, 0, 1) at (0, 0, 8)
extrude "Extrude6" add sketch "bow" against normal blind 2.2 contours L3 L4 L5 L6 L7 L8 L9 bodies 1 2
move_face "OffsetFaces1" offset -0.125 2 faces at (-0.2, 4.3858, 8.75) (-0.2, -18.2808, 0.75) on bodies 1
equation "Single1 = 1 mm"
equation "Single2 = 1 mm"
equation "Single3 = 1 mm"
equation "Single4 = 1 mm"
equation "Single5 = 1 mm"
equation "Single6 = 1 mm"
equation "Double1 = 1 mm"
equation "Double2 = 1 mm"
equation "Double3 = 1 mm"
equation "Double4 = 1 mm"
equation "Double5 = 1 mm"
equation "Double6 = 1 mm"
equation "TrackToleranceAdd = 0 mm"
equation "d21 = d20"
equation "d22 = d20"
equation "d23 = d20"
equation "d24 = d20"
equation "d25 = d20"
equation "d26 = 1.5 mm + 0.5 * Single1"
equation "d27 = 1.5 mm + 0.5 * Single2"
equation "d28 = 1.5 mm + 0.5 * Single3"
equation "d29 = 1.5 mm + 0.5 * Single4"
equation "d30 = 1.5 mm + 0.5 * Single5"
equation "d31 = 1.5 mm + 0.5 * Single6"
equation "d32 = 1.2 mm + TrackToleranceAdd"
equation "d33 = d32"
equation "d34 = d32"
equation "d35 = d32"
equation "d36 = d32"
equation "d37 = d32"
equation "d38 = 0.3 mm + 0.5 * TrackToleranceAdd"
equation "d39 = d38"
equation "d40 = d38"
equation "d41 = d38"
equation "d42 = d38"
equation "d43 = d38"
equation "d44 = d38"
equation "d45 = d38"
equation "d46 = d38"
equation "d47 = d38"
equation "d48 = d38"
equation "d49 = d38"
equation "d50 = 0.5 * d32"
equation "d51 = d50"
equation "d54 = d20"
equation "d55 = d20"
equation "d56 = d20"
equation "d57 = d20"
equation "d58 = d20"
equation "d59 = d20"
equation "d60 = 2 mm + 0.5 * Double1"
equation "d61 = 2 mm + 0.5 * Double2"
equation "d62 = 2 mm + 0.5 * Double3"
equation "d63 = 2 mm + 0.5 * Double4"
equation "d64 = 2 mm + 0.5 * Double5"
equation "d65 = 2 mm + 0.5 * Double6"
equation "d67 = d66"
equation "d68 = d66"
equation "d69 = d66"
equation "d70 = d66"
equation "d71 = d66"
equation "d72 = d66"
equation "d73 = d66"
equation "d74 = d66"
equation "d75 = d66"
equation "WiderTrack = 1.7 mm + TrackToleranceAdd"
equation "d77 = d66 - ( 0.5 * d32 ) + ( 0.5 * WiderTrack )"
equation "d78 = d77"
equation "d79 = d32"
equation "d80 = d32"
equation "d81 = d32"
equation "d82 = d32"
equation "d83 = d32"
equation "d84 = d32"
equation "d85 = d32"
equation "d86 = d32"
equation "d87 = d32"
equation "d88 = d32"
equation "d89 = WiderTrack"
equation "d90 = d89"
equation "d91 = d38"
equation "d92 = d38"
equation "d93 = d38"
equation "d94 = d38"
equation "d95 = d38"
equation "d96 = d38"
equation "d97 = d38"
equation "d98 = d38"
equation "d99 = d38"
equation "d100 = d38"
equation "d101 = d38"
equation "d102 = d77"
equation "d103 = d77"
equation "d104 = d38"
equation "d105 = d38"
equation "d106 = d38"
equation "d107 = d38"
equation "d108 = d38"
equation "d109 = d38"
equation "d110 = d38"
equation "d111 = d38"
equation "d112 = d38"
equation "d113 = d38"
equation "d114 = d38"
equation "d115 = d38"
equation "d116 = d38"
equation "d118 = d66"
equation "d119 = d117"
equation "d120 = d66"
equation "d121 = d50"
equation "d122 = d50"
equation "d123 = d50"
equation "d124 = d50"
equation "d125 = 0.5 * d52"
equation "d126 = d125"
equation "d127 = d19 + ( d20 * 4 )"
equation "d128 = d20"
equation "d129 = d20"
equation "d130 = d64"
equation "d131 = d65"
equation "d132 = d66"
equation "d133 = d66"
equation "d134 = 0.5 * d32"
equation "d135 = d134"
equation "d136 = d134"
equation "d137 = d134"
equation "d138 = d134"
equation "d139 = d134"
equation "d140 = d38"
equation "d141 = d38"
equation "d142 = d38"
equation "d143 = d38"
equation "d144 = d77"
equation "d145 = d77"
equation "d147 = 2 * ( 0.5 * ( WiderTrack - d32 ) ) * sin(45 deg)"
equation "d148 = d146"
equation "d149 = d147"
equation "d150 = 0.25 * d19"
equation "d151 = d146"
equation "d152 = d147"
equation "d153 = d146"
equation "d154 = d147"
equation "d155 = d150"
equation "d156 = d134"
equation "d162 = d38"
equation "d165 = d77"
equation "d166 = d77"
equation "d167 = d38"
equation "d168 = d38"
equation "d169 = d117"
equation "d170 = d77"
equation "d171 = d77"
equation "d172 = d134"
equation "d173 = d134"
equation "d174 = d134"
equation "d175 = d38"
equation "d176 = 0.25 * WiderTrack"
equation "d177 = 0.5 * ( WiderTrack - d32 )"
equation "d178 = d134"
equation "d179 = d134"
equation "d180 = d134"
equation "d181 = d134"
equation "d182 = d38"
equation "d183 = d38"
equation "d184 = 0.25 * WiderTrack"
equation "d185 = 0.5 * ( WiderTrack - d32 )"
equation "d186 = d117"
equation "d187 = d77"
equation "d188 = d77"
equation "d190 = 0.5 * WiderTrack"
equation "d191 = d190"
equation "d192 = d190"
equation "d193 = d190"
equation "d194 = d125"
equation "d195 = d125"
equation "d202 = 2.5 mm - d201"
equation "d204 = d202"
equation "d205 = d201"
equation "d206 = d202"
equation "d207 = d203"
equation "d208 = d202"
equation "d210 = d66"
equation "d211 = d66"
equation "d212 = d38"
equation "d213 = d38"
equation "d215 = d214"
named bodies: "blade", "blade (1)"
